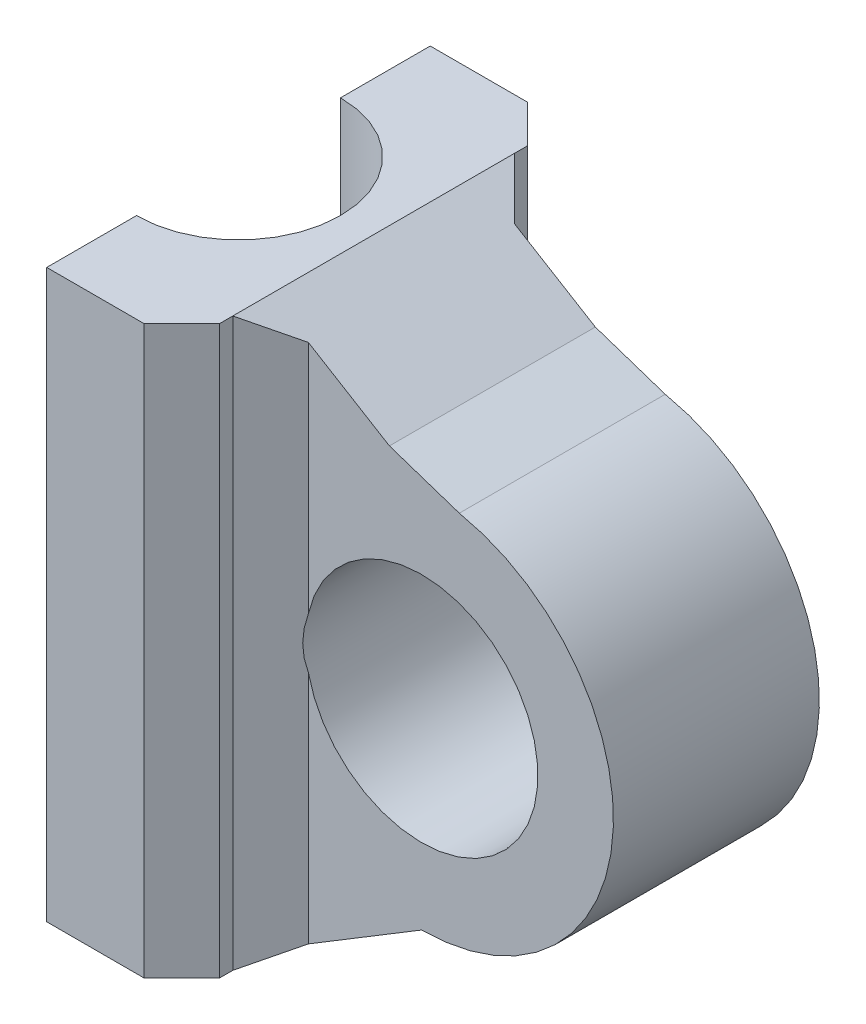
# Autodesk Inventor part: rack-mounts
Saved by Autodesk Inventor 2024.1 (Build 281209000, 209)
## iProperties
Created: 2025-08-22
Part Number: rack-mounts
Material: Generic
Document SubType Name: Modeling
Designer: iwheard
Density: 1 g/cm^3
Appearance: Default
Author: iwheard
Autodesk Inventor part; units mm, degrees
ref_plane "YZ Plane" through (0, 0, 0) normal (1, 0, 0) x (0, 1, 0)
ref_plane "XZ Plane" through (0, 0, 0) normal (0, 1, 0) x (-1, 0, 0)
ref_plane "Work Plane1" through (0, 0, 52.5) normal (0, 0, 1) x (1, 0, 0)
ref_plane "Work Plane2" through (0, 240, 52.5) normal (0, -1, 0) x (0, 0, -1)
sketch "Sketch2" plane through (0, 240, 52.5) normal (0, -1, 0) x (0, 0, -1)
  circle A0 centre (0, 0) radius 5.15 projected
  line L0 (-10.15, 7.15) -> (10.15, 7.15)
  line L1 (10.15, 7.15) -> (10.15, 0)
  line L2 (10.15, 0) -> (-10.15, 0)
  line L3 (-10.15, 0) -> (-10.15, 7.15)
  line L4 (-5.15, 5.15) -> (5.15, 5.15) construction
  line L5 (5.15, 5.15) -> (5.15, -5.15) construction
  line L6 (5.15, -5.15) -> (-5.15, -5.15) construction
  line L7 (-5.15, -5.15) -> (-5.15, 5.15) construction
  circle A1 centre (0, 0) radius 5.4
  point P0 (52.5, 0)
  point P1 (-5.15, 0)
  point P2 (5.15, 0)
  point P3 (-5.4, 0)
  point P4 (5.4, 0)
  dimension "d0" = 5
  dimension "d1" = 5
  dimension "d2" = 2
  dimension "d5" = 0.25
  constraints: 16 end point, 4 tangent, 1 centre point, 1 coincident, 1 horizontal, 1 midpoint
  measures "d0" distance between parallel lines of L1 L5
  measures "d1" distance between parallel lines of L3 L7
  measures "d2" distance between parallel lines of L0 L4
  measures "d5" radial gap between concentric circles of A1 A0
extrude "Extrusion1" add sketch "Sketch2" against normal blind 30 contours A1 L2 L3 L0 L1
sketch "Sketch3" plane through (0, 240, 62.65) normal (0, 0, 1) x (1, 0, 0)
  line L0 (7.15, 30) -> (15.15, 25.15)
  line L1 (15.15, 4.85) -> (7.15, 0)
  circle A0 centre (15.15, 15) radius 6.15
  line L2 (7.15, 0) -> (7.15, 30) projected
  line L3 (0, 30) -> (7.15, 30) projected
  circle A1 centre (15.15, 15) radius 10.15
  point P0 (0, -240)
  point P1 (33.3346, 15)
  point P2 (7.15, 15)
  dimension "d6" = 12.3
  dimension "d7" = 8
  dimension "d8" = 15
  dimension "d9" = 4
  constraints: 4 end point, 2 centre point, 2 point on circle, 2 vertical alignment, 1 coincident, 1 concentric, 1 horizontal alignment
  measures "d6" diameter of A0
  measures "d7" distance from line of L2 A0.centre
  measures "d8" distance from line of A0.centre L3
  measures "d9" radial gap between concentric circles of A1 A0
extrude "Extrusion2" add sketch "Sketch3" against normal up to surface (20.3 mm away) contours L0 A1 L2 | A1 L2 | A1 L1 L2 picked at (7.7667, 15)
sketch "Sketch4" plane through (0, 240, 52.5) normal (0, -1, 0) x (1, 0, 0)
  line L0 (25.3, 10.15) -> (25.3, -10.15) projected
  line L1 (25.3, 5.45) -> (7.15, 5.45)
  line L2 (7.15, 5.45) -> (7.15, -5.45)
  line L3 (7.15, -5.45) -> (25.3, -5.45)
  line L4 (25.3, -5.45) -> (25.3, 5.45)
  line L5 (7.15, 10.15) -> (0, 10.15) projected
  line L6 (0, -10.15) -> (7.15, -10.15) projected
  line L7 (15.15, -10.15) -> (15.15, -10.15) projected
  line L8 (15.15, 10.15) -> (15.15, -10.15) projected
  line L9 (15.15, 10.15) -> (15.15, 10.15) projected
  line L10 (15.15, 10.15) -> (15.15, -10.15) projected
  line L11 (7.15, -10.15) -> (15.15, -10.15) projected
  line L12 (15.15, 10.15) -> (15.15, -10.15) projected
  line L13 (7.15, 10.15) -> (15.15, 10.15) projected
  line L14 (7.15, -10.15) -> (7.15, 10.15) projected
  line L15 (7.15, -10.15) -> (7.15, 10.15) projected
  line L16 (7.15, 10.15) -> (0, 10.15) projected
  line L17 (0, 10.15) -> (0, 5.4) projected
  arc A0 (0, -5.4) -> (0, 5.4) centre (0, 0) ccw projected
  line L18 (0, -5.4) -> (0, -10.15) projected
  line L19 (0, -10.15) -> (7.15, -10.15) projected
  line L20 (25.3, 10.15) -> (15.15, 10.15) projected
  line L21 (25.3, -10.15) -> (15.15, -10.15) projected
  point P0 (0, -52.5)
  point P1 (25.3, -5.45)
  point P2 (7.15, -5.45)
  point P3 (7.15, 5.45)
  point P4 (25.3, 5.45)
  dimension "d14" = 4.7
  dimension "d15" = 4.7
  constraints: 8 end point
  measures "d14" distance between parallel lines of L1 L5
  measures "d15" distance between parallel lines of L6 L3
extrude "Extrusion3" cut sketch "Sketch4" against normal through all contours L0 L1 L8 L20 | L8 L1 L14 L13 | L0 L21 L8 L3 | L8 L11 L14 L3
chamfer "Chamfer1" distance 2 angle 45 5 edges at (7.15, 255, 47.05) (7.15, 255, 57.95) (15.15, 265.15, 52.5) (7.15, 255, 62.65) (7.15, 255, 42.35)
body "Solid1"
